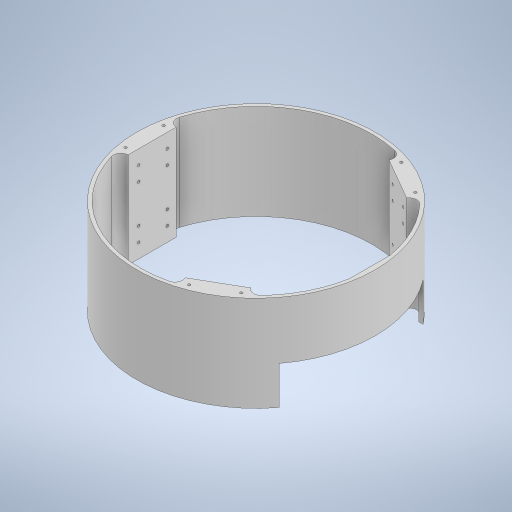
# Autodesk Inventor part: allwall
Saved by Autodesk Inventor 2023 (Build 270158000, 158)
## iProperties
Created: 2022-12-04
Part Number: allwall
Material: 一般
Document SubType Name: Modeling
Designer: RiSA
Density: 1 g/cm^3
Appearance: 既定
Author: RiSA
Autodesk Inventor part; units mm, degrees
ref_plane "YZ Plane" through (0, 0, 0) normal (1, 0, 0) x (0, 1, 0)
ref_plane "XZ Plane" through (0, 0, 0) normal (0, 1, 0) x (-1, 0, 0)
ref_plane "XY Plane" through (0, 0, 0) normal (0, 0, 1) x (1, 0, 0)
sketch "スケッチ1" plane through (0, 0, 0) normal (0, 1, 0) x (-1, 0, 0)
  circle A0 centre (0, 0) radius 125
  circle A1 centre (0, 0) radius 121.5
  line L0 (118.86, 0) -> (118.86, -25.1903)
  line L1 (118.86, 0) -> (118.86, 25.1903)
  line L2 (118.86, 25.1903) -> (108.86, 25.1903)
  line L3 (108.86, 25.1903) -> (108.86, -25.1903)
  line L4 (108.86, -25.1903) -> (118.86, -25.1903)
  line L5 (118.86, -25.1903) -> (118.86, 25.1903)
  line L6 (-59.43, 102.9358) -> (-37.6146, 115.5309)
  line L7 (-59.43, 102.9358) -> (-81.2454, 90.3406)
  line L8 (-81.2454, 90.3406) -> (-76.2454, 81.6804)
  line L9 (-76.2454, 81.6804) -> (-32.6146, 106.8707)
  line L10 (-32.6146, 106.8707) -> (-37.6146, 115.5309)
  line L11 (-37.6146, 115.5309) -> (-81.2454, 90.3406)
  line L12 (-59.43, -102.9358) -> (-81.2454, -90.3406)
  line L13 (-59.43, -102.9358) -> (-37.6146, -115.5309)
  line L14 (-37.6146, -115.5309) -> (-32.6146, -106.8707)
  line L15 (-32.6146, -106.8707) -> (-76.2454, -81.6804)
  line L16 (-76.2454, -81.6804) -> (-81.2454, -90.3406)
  line L17 (-81.2454, -90.3406) -> (-37.6146, -115.5309)
  dimension "d0" = 250
  dimension "d1" = 243
  dimension "d2" = 118.86
  dimension "d3" = 10
  dimension "d6" = 360
  constraints: 36 end point, 3 point on line, 2 centre point, 2 coincident, 2 parallel, 2 point on circle, 1 horizontal, 1 perpendicular, 1 vertical, 37 other
  measures "d0" diameter of A0
  measures "d1" diameter of A1
  measures "d2" distance of A1.centre L0.start
  measures "d3" distance of L4.end L3.end
extrude "押し出し1" add sketch "スケッチ1" along normal blind 100 contours A0 | A1 L0 L1 | L1 L0 L4 L3 L2 | L6 L7 A1 | L10 L9 L8 L7 L6 | A1 L12 L13 | L13 L12 L16 L15 L14
fillet "フィレット1" radius 8 6 edges at (37.6146, 50, -115.5309) (81.2454, 50, -90.3406) (-118.86, 50, 25.1903) (-118.86, 50, -25.1903) (81.2454, 50, 90.3406) (37.6146, 50, 115.5309)
sketch "スケッチ4" plane through (0, 100, 0) normal (0, 1, 0) x (1, 0, 0)
  line L0 (119.6242, 0) -> (119.6242, -21.2671)
  arc A0 (88.8593, -82.863) -> (88.8593, 82.863) centre (0, 0) ccw projected
  line L1 (119.6242, 0) -> (119.6242, 21.2671)
  arc A1 (119.6242, -21.2671) -> (119.6242, 21.2671) centre (0, 0) ccw
  constraints: 4 end point, 4 point on circle, 1 centre point, 1 point on line, 1 vertical
extrude "押し出し4" add sketch "スケッチ4" against normal blind 100
sketch "スケッチ5" plane through (119.6242, 100, -21.2671) normal (-1, 0, 0) x (0, 0, 1)
  line L0 (96.7671, -100) -> (-54.2329, -100)
  line L1 (-54.2329, -100) -> (-54.2329, -64.5)
  line L2 (-54.2329, -64.5) -> (96.7671, -64.5)
  line L3 (96.7671, -64.5) -> (96.7671, -100)
  line L4 (96.7671, -100) -> (-54.2329, -64.5) construction
  line L5 (-54.2329, -100) -> (96.7671, -64.5) construction
  line L6 (42.5342, -100) -> (0, -100) projected
  point P0 (21.2671, -100)
  point P1 (21.2671, -82.25)
  dimension "d20" = 151
  dimension "d21" = 35.5
  dimension "d22" = 0
  constraints: 12 end point, 2 midpoint, 2 parallel, 1 horizontal, 1 perpendicular
  measures "d20" distance of L1.end L2.end
  measures "d21" distance of L0.end L1.end
  measures "d22" distance between parallel lines of L6 L0
extrude "押し出し5" add sketch "スケッチ5" along normal blind 30
sketch "スケッチ6" plane through (89.6242, 100, -21.2671) normal (-1, 0, 0) x (0, 0, 1)
  line L0 (96.7671, -64.5) -> (-54.2329, -64.5) projected
  line L1 (-54.2329, -100) -> (96.7671, -100) projected
  line L2 (-54.2329, -64.5) -> (96.7671, -64.5)
  line L3 (96.7671, -64.5) -> (96.7671, -100)
  line L4 (96.7671, -100) -> (-54.2329, -100)
  line L5 (-54.2329, -100) -> (-54.2329, -64.5)
  line L6 (-54.2329, -64.5) -> (-54.2329, -100) projected
  line L7 (-54.2329, -64.5) -> (96.7671, -64.5)
  line L8 (96.7671, -64.5) -> (96.7671, -60)
  line L9 (96.7671, -60) -> (-54.2329, -60)
  line L10 (-54.2329, -60) -> (-54.2329, -64.5)
  point P0 (21.2671, -100)
  point P1 (-54.2329, -100)
  dimension "d27" = 151
  dimension "d28" = 4.5
  constraints: 16 end point, 4 parallel, 2 horizontal, 2 perpendicular
  measures "d27" distance of L9.end L8.end
  measures "d28" distance of L8.end L7.end
extrude "押し出し6" cut sketch "スケッチ6" against normal blind 100
sketch "スケッチ7" plane through (-108.86, 0, 25.1903) normal (1, 0, 0) x (0, 0, -1)
  line L0 (0, 100) -> (50.3806, 100) projected
  line L1 (50.3806, 0) -> (50.3806, 100) projected
  line L2 (50.3806, 50) -> (0, 50)
  line L3 (0, 0) -> (0, 100) projected
  point P0 (25.1903, 0)
  point P1 (41.0542, 85)
  point P2 (26.0542, 85)
  point P3 (11.0542, 85)
  point P4 (11.0542, 70)
  point P5 (41.0542, 70)
  point P6 (41.0542, 15)
  point P7 (11.0542, 15)
  point P8 (11.0542, 30)
  point P9 (41.0542, 30)
  dimension "d29" = 15
  dimension "d30" = 15
  dimension "d31" = 15
  dimension "d32" = 15
  dimension "d33" = 15
  constraints: 4 symmetric about line, 2 end point, 2 midpoint
  measures "d29" distance from line of point (41.054, 85) L0
  measures "d30" distance of point (26.054, 85) point (11.054, 85)
  measures "d31" distance of point (41.054, 85) point (26.054, 85)
  measures "d32" distance from line of L0 point (26.054, 85)
  measures "d33" distance of point (11.054, 70) point (11.054, 85)
hole "穴1" at (-108.86, 85, -15.864) at (-108.86, 85, 14.136) at (-108.86, 70, 14.136) at (-108.86, 70, -15.864) at (-108.86, 30, 14.136) at (-108.86, 30, -15.864) at (-108.86, 15, -15.864) at (-108.86, 15, 14.136) direction (-1, 0, 0) diameter 2.7 depth 10 tip angle 118
sketch "スケッチ8" plane through (76.2454, 0, -81.6804) normal (-0.5, 0, 0.8660254) x (0.8660254, 0, 0.5)
  line L0 (-50.3806, 100) -> (0, 100) projected
  line L1 (0, 0) -> (0, 100) projected
  line L2 (0, 50) -> (-50.3806, 50)
  line L3 (-50.3806, 0) -> (-50.3806, 100) projected
  point P0 (-25.1903, 0)
  point P1 (-25.1903, 85)
  point P2 (-10.1903, 84.8886)
  point P3 (-40.1903, 84.8886)
  point P4 (-40.1903, 69.8886)
  point P5 (-10.1903, 69.8886)
  point P6 (-10.1903, 15.1114)
  point P7 (-40.1903, 15.1114)
  point P8 (-40.1903, 30.1114)
  point P9 (-10.1903, 30.1114)
  dimension "d41" = 15
  dimension "d42" = 15
  dimension "d43" = 15
  dimension "d44" = 15
  constraints: 4 symmetric about line, 2 end point, 2 midpoint
  measures "d41" distance from line of point (-25.19, 85) L0
  measures "d42" horizontal distance of point (-10.19, 84.889) point (-25.19, 85)
  measures "d43" horizontal distance of point (-40.19, 84.889) point (-25.19, 85)
  measures "d44" distance of point (-40.19, 69.889) point (-40.19, 84.889)
hole "穴2" at (67.4204, 84.8886, -86.7755) at (41.4396, 84.8886, -101.7755) at (41.4396, 69.8886, -101.7755) at (67.4204, 69.8886, -86.7755) at (41.4396, 15.1114, -101.7755) at (41.4396, 30.1114, -101.7755) at (67.4204, 30.1114, -86.7755) at (67.4204, 15.1114, -86.7755) direction (0.5, 0, -0.8660254) diameter 2.7 depth 10 tip angle 118
sketch "スケッチ9" plane through (32.6146, 0, 106.8707) normal (-0.5, 0, -0.8660254) x (-0.8660254, 0, 0.5)
  line L0 (-50.3806, 100) -> (0, 100) projected
  line L1 (0, 0) -> (0, 100) projected
  line L2 (0, 50) -> (-21.724, 50)
  point P0 (-25.1903, 0)
  point P1 (-40.3552, 85)
  point P2 (-25.3552, 85)
  point P3 (-10.3552, 85)
  point P4 (-40.3552, 70)
  point P5 (-10.3552, 70)
  point P6 (-40.3552, 15)
  point P7 (-10.3552, 15)
  point P8 (-40.3552, 30)
  point P9 (-10.3552, 30)
  dimension "d52" = 15
  dimension "d53" = 15
  dimension "d54" = 15
  dimension "d55" = 15
  dimension "d56" = 15
  constraints: 4 symmetric about line, 2 end point, 1 horizontal, 1 midpoint
  measures "d52" distance from line of point (-25.355, 85) L0
  measures "d53" distance from line of point (-40.355, 85) L0
  measures "d54" distance of point (-25.355, 85) point (-40.355, 85)
  measures "d55" distance of point (-10.355, 85) point (-25.355, 85)
  measures "d56" distance of point (-40.355, 70) point (-40.355, 85)
hole "穴3" at (67.5632, 85, 86.6931) at (41.5824, 85, 101.6931) at (67.5632, 70, 86.6931) at (41.5824, 70, 101.6931) at (67.5632, 15, 86.6931) at (67.5632, 30, 86.6931) at (41.5824, 30, 101.6931) at (41.5824, 15, 101.6931) direction (0.5, 0, 0.8660254) diameter 2.7 depth 10 tip angle 118
sketch "スケッチ10" plane through (0, 100, 0) normal (0, 1, 0) x (1, 0, 0)
  line L0 (-108.86, -25.1903) -> (-108.86, 25.1903) projected
  point P0 (0, 0)
  point P1 (-116.86, 0)
  point P2 (-116.86, -20)
  point P3 (-116.86, 20)
  point P4 (41.1095, -111.2037)
  point P5 (75.7505, -91.2037)
  point P6 (58.43, -101.2037)
  point P7 (75.7505, 91.2037)
  point P8 (41.1095, 111.2037)
  point P9 (58.43, 101.2037)
  dimension "d64" = 8
  dimension "d65" = 20
  dimension "d66" = 20
  dimension "d76" = 360
  constraints: 10 other
  measures "d64" distance from line of L0 point (-116.86, 0)
  measures "d65" distance of point (-116.86, 0) point (-116.86, -20)
  measures "d66" distance of point (-116.86, 0) point (-116.86, 20)
hole "穴4" at (-116.86, 100, 20) at (-116.86, 100, -20) at (75.7505, 100, 91.2037) at (41.1095, 100, 111.2037) at (41.1095, 100, -111.2037) at (75.7505, 100, -91.2037) direction (0, -1, 0) diameter 2.7 depth 10
sketch "スケッチ11" plane through (0, 0, 0) normal (0, -1, 0) x (1, 0, 0)
  circle A0 centre (-116.86, 0) radius 1.35 projected
  circle A1 centre (-116.86, -20) radius 1.35 projected
  circle A2 centre (-116.86, 20) radius 1.35 projected
  point P0 (0, 0)
  point P1 (41.1095, -111.2037)
  point P2 (75.7505, -91.2037)
  point P3 (58.43, -101.2037)
  point P4 (75.7505, 91.2037)
  point P5 (41.1095, 111.2037)
  point P6 (58.43, 101.2037)
  dimension "d80" = 360
  constraints: 3 coincident, 10 other
hole "穴5" at (-116.86, 0, -20) at (-116.86, 0, 20) at (41.1095, 0, -111.2037) at (75.7505, 0, -91.2037) at (75.7505, 0, 91.2037) at (41.1095, 0, 111.2037) direction (0, 1, 0) diameter 2.7 depth 10
